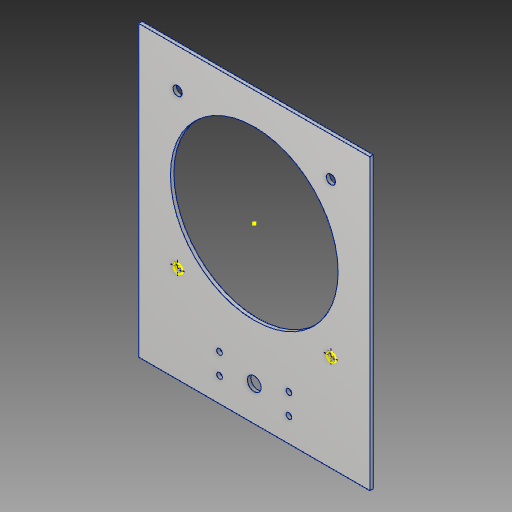
# Autodesk Inventor part: ベアリング板
Saved by Autodesk Inventor 2019 (Build 230136000, 136)
## iProperties
Created: 2020-10-01
Part Number: ベアリング板
Material: アルミニウム 6061
Document SubType Name: Modeling
Designer: Toshihito
Density: 2.7 g/cm^3
Appearance: アルミニウム - フラット
Author: Toshihito
Autodesk Inventor part; units mm, degrees
ref_plane "YZ Plane" through (0, 0, 0) normal (1, 0, 0) x (0, 1, 0)
ref_plane "XZ Plane" through (0, 0, 0) normal (0, 1, 0) x (-1, 0, 0)
ref_plane "XY Plane" through (0, 0, 0) normal (0, 0, 1) x (1, 0, 0)
sketch "スケッチ1" plane through (0, 0, 0) normal (0, 0, 1) x (1, 0, 0)
  line L0 (-100, 100) -> (100, 100)
  line L1 (100, 100) -> (100, -100)
  line L2 (100, -100) -> (-100, -100)
  line L3 (-100, -100) -> (-100, 100)
  line L4 (-100, 100) -> (100, -100) construction
  line L5 (100, 100) -> (-100, -100) construction
  circle A0 centre (0, 0) radius 93.75 construction
  circle A1 centre (-66.2913, 66.2913) radius 4
  circle A2 centre (66.2913, 66.2913) radius 4
  circle A3 centre (66.2913, -66.2913) radius 4
  circle A4 centre (-66.2913, -66.2913) radius 4
  dimension "d0" = 200
  dimension "d1" = 200
  dimension "d2" = 187.5
  dimension "d3" = 8
  dimension "d4" = 8
  dimension "d5" = 8
  dimension "d6" = 8
  constraints: 12 end point, 5 centre point, 4 point on circle, 4 point on line, 2 midpoint, 2 parallel, 1 coincident, 1 horizontal, 1 perpendicular
  measures "d0" distance of L1.end L2.end
  measures "d1" distance of L0.end L1.end
  measures "d2" diameter of A0
  measures "d3" diameter of A1
  measures "d4" diameter of A2
  measures "d5" diameter of A3
  measures "d6" diameter of A4
extrude "押し出し1" add sketch "スケッチ1" along normal blind 3
sketch "スケッチ2" plane through (0, 0, 0) normal (0, 0, -1) x (-1, 0, 0)
  circle A0 centre (0, 0) radius 72.5
  dimension "d9" = 145
  constraints: 1 centre point, 1 coincident
  measures "d9" diameter of A0
extrude "押し出し2" cut sketch "スケッチ2" against normal blind 10
sketch "スケッチ3" plane through (0, 0, 3) normal (0, 0, 1) x (1, 0, 0)
  circle A0 centre (-66.2913, -66.2913) radius 4 projected
  circle A1 centre (66.2913, -66.2913) radius 4 projected
  point P0 (0, 0)
  constraints: 2 coincident
sketch "スケッチ4" plane through (-100, -100, 0) normal (0, -1, 0) x (1, 0, 0)
  line L0 (0, 0) -> (0, 3) projected
  line L1 (200, 0) -> (200, 3) projected
  line L2 (0, 3) -> (200, 3)
  line L3 (200, 3) -> (200, 0)
  line L4 (200, 0) -> (0, 0)
  line L5 (0, 0) -> (0, 3)
  point P0 (100, 0)
  constraints: 8 end point, 2 parallel, 1 horizontal, 1 perpendicular
extrude "押し出し3" add sketch "スケッチ4" along normal blind 50
sketch "スケッチ5" plane through (0, 0, 3) normal (0, 0, 1) x (1, 0, 0)
  circle A0 centre (0, -120) radius 6
  point P0 (0, 0)
  dimension "d14" = 12
  constraints: 1 centre point
  measures "d14" diameter of A0
extrude "押し出し4" cut sketch "スケッチ5" against normal blind 100
sketch "スケッチ6" plane through (0, 0, 3) normal (0, 0, 1) x (1, 0, 0)
  circle A0 centre (0, -120) radius 6 projected
  line L0 (0, -120) -> (-30, -120)
  line L1 (-30, -120) -> (30, -120)
  line L2 (30, -120) -> (30, -111)
  line L3 (30, -111) -> (30, -129)
  line L4 (30, -129) -> (-30, -111)
  line L5 (-30, -111) -> (-30, -129)
  circle A1 centre (-30, -111) radius 2.5
  circle A2 centre (-30, -129) radius 2.5
  circle A3 centre (30, -111) radius 2.5
  circle A4 centre (30, -129) radius 2.5
  point P0 (0, 0)
  dimension "d17" = 30
  dimension "d18" = 60
  dimension "d19" = 9
  dimension "d20" = 90
  dimension "d21" = 18
  dimension "d22" = 5
  dimension "d23" = 5
  dimension "d24" = 5
  dimension "d25" = 5
  constraints: 12 end point, 4 centre point, 4 coincident, 2 perpendicular, 2 point on line, 1 horizontal
  measures "d17" distance of L0.start L0.end
  measures "d18" distance of L0.end L1.end
  measures "d19" distance of L1.end L2.end
  measures "d20" angle of L2 L1
  measures "d21" distance of L2.end L3.end
  measures "d22" diameter of A1
  measures "d23" diameter of A2
  measures "d24" diameter of A3
  measures "d25" diameter of A4
extrude "押し出し5" cut sketch "スケッチ6" against normal blind 100 contours A3 | A2 | A1 L5 L4 | L4 L5 A1 | A4 L3 L4 | L4 L3 A4
